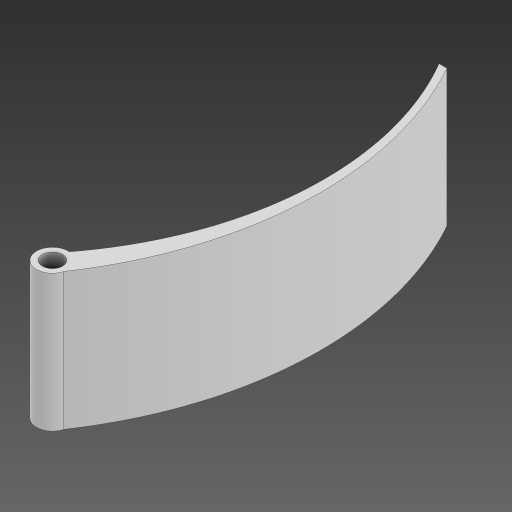
# Autodesk Inventor part: protect
Saved by Autodesk Inventor 2023 (Build 270158000, 158)
## iProperties
Created: 2025-06-27
Part Number: protect
Material: Типовые
Document SubType Name: Modeling
Designer: daa
Density: 1 g/cm^3
Appearance: По умолчанию
Author: daa
Autodesk Inventor part; units mm, degrees
ref_plane "YZ Plane" through (0, 0, 0) normal (1, 0, 0) x (0, 1, 0)
ref_plane "XZ Plane" through (0, 0, 0) normal (0, 1, 0) x (-1, 0, 0)
ref_plane "XY Plane" through (0, 0, 0) normal (0, 0, 1) x (1, 0, 0)
sketch "Эскиз1" plane through (0, 0, 0) normal (0, 1, 0) x (-1, 0, 0)
  circle A0 centre (-56.8828, 132.85) radius 1.5
  circle A1 centre (-56.8828, 132.85) radius 1.5
  circle A2 centre (-56.8828, 132.85) radius 2.6
  line L0 (-62.783, 39.7675) -> (-64.783, 39.7675)
  circle A3 centre (-56.8828, 132.85) radius 4.0649
  line L1 (-60.8228, 133.85) -> (-52.9427, 133.85)
  arc A4 (-60.8228, 133.85) -> (-64.783, 39.7675) centre (13.8313, 83.583) ccw
  arc A5 (-57.163, 128.7948) -> (-62.783, 39.7675) centre (6.3077, 80.097) ccw
  point P0 (-68.2724, 116.2724)
  point P1 (-62.783, 39.7675)
  dimension "d26" = 3
  dimension "d27" = 5.2
  dimension "d28" = 2
  dimension "d29" = 90
  dimension "d30" = 80
  dimension "d31" = 93.0825
  dimension "d32" = 7.9002
  constraints: 7 point on circle, 6 centre point, 4 end point, 3 coincident, 1 concentric, 1 horizontal
  measures "d26" diameter of A0
  measures "d27" diameter of A2
  measures "d28" distance of L0.start L0.end
  measures "d29" radius of A4
  measures "d30" radius of A5
  measures "d31" vertical distance of A3.centre L0.start
  measures "d32" horizontal distance of A0.centre L0.end
extrude "Выдавливание1" add sketch "Эскиз1" along normal blind 35 contours L1 A3 A2 | A2 L1 A3 | A3 A5 L0 A4
